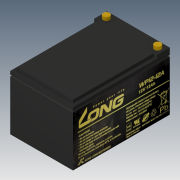
# Autodesk Inventor part: 800-10-ELECTRONICS-BATTERY-12V-12Ah
Saved by Autodesk Inventor 2018.2 (Build 222227000, 227)
## iProperties
Manager: feesmrt
Company: FRANC0R
Created: 2017-12-05
Part Number: 800-10-ELECTRONICS-BATTERY-12V-12Ah
Material: ABS-Kunststoff
Document SubType Name: Modeling
Designer: feesmrt
Density: 1.06 g/cm^3
Appearance: Glatt - schwarz
Project: Rescue Robot
Cost Center: -
Engineer: feesmrt
Authority: feesmrt
Description: Lead-Acid Battery WP12-12 12V 12Ah
Stock Number: 800-10-ELECTRONICS-BATTERY-12V-12Ah
Catalog Web Link: Reichelt
Vendor: https://www.reichelt.de/Blei-Vlies-Akkus-12V-Kung-Long/WP-12-12/3/index.html?ACTION=3&GROUPID=4232&ARTICLE=44421&START=0&OFFSET
Author: feesmrt
Subject: Rescue Robot
Title: Lead-Acid Battery WP12-12 12V 12Ah
Revision Number: 1
Autodesk Inventor part; units mm, degrees
ref_plane "YZ Plane" through (0, 0, 0) normal (1, 0, 0) x (0, 1, 0)
ref_plane "XZ Plane" through (0, 0, 0) normal (0, 1, 0) x (-1, 0, 0)
ref_plane "XY Plane" through (0, 0, 0) normal (0, 0, 1) x (1, 0, 0)
sketch "Skizze1" plane through (0, 0, 0) normal (0, 0, 1) x (1, 0, 0)
  line L0 (-49, -75.5) -> (49, -75.5)
  line L1 (49, -75.5) -> (49, 75.5)
  line L2 (49, 75.5) -> (-49, 75.5)
  line L3 (-49, 75.5) -> (-49, -75.5)
  line L4 (-49, -75.5) -> (49, 75.5) construction
  line L5 (49, -75.5) -> (-49, 75.5) construction
  point P0 (0, 0)
  dimension "d0" = 98
  dimension "d1" = 151
  constraints: 12 end point, 2 midpoint, 2 parallel, 1 horizontal, 1 perpendicular
  measures "d0" distance of L1.end L2.end
  measures "d1" distance of L0.end L1.end
extrude "Grundkörper" add sketch "Skizze1" along normal blind 83
chamfer "Fase" distance 2.5 angle 45 8 edges at (-49, 0, 83) (0, -75.5, 83) (49, 0, 83) (0, 75.5, 83) (0, -75.5, 0) (-49, 0, 0) (49, 0, 0) (0, 75.5, 0)
sketch "Skizze2" plane through (0, 0, 83) normal (0, 0, 1) x (1, 0, 0)
  line L0 (49, -75.5) -> (49, 75.5) projected
  line L1 (49, 75.5) -> (-49, 75.5) projected
  line L2 (-49, -75.5) -> (49, -75.5) projected
  line L3 (-49, 75.5) -> (-49, -75.5) projected
  point P0 (0, 0)
extrude "Cap" add sketch "Skizze2" along normal blind 10
sketch "Skizze3" plane through (0, 0, 93) normal (0, 0, 1) x (1, 0, 0)
  line L0 (44, 55.5) -> (-44, 55.5)
  line L1 (-44, 55.5) -> (-44, -70.5)
  line L2 (-44, -70.5) -> (44, -70.5)
  line L3 (44, -70.5) -> (44, 55.5)
  line L4 (0, 105.7) -> (0, -105.7) construction
  line L5 (49, -75.5) -> (49, 75.5) projected
  line L6 (-49, -75.5) -> (49, -75.5) projected
  line L7 (44, 55.5) -> (49, 55.5)
  line L8 (49, -75.5) -> (49, 75.5) projected
  line L9 (49, 55.5) -> (49, -75.5)
  line L10 (-49, 75.5) -> (-49, -75.5) projected
  line L11 (49, -75.5) -> (-49, -75.5)
  line L12 (-49, -75.5) -> (-49, 55.5)
  line L13 (-44, 55.5) -> (-49, 55.5)
  line L14 (-46.5, -73) -> (-46.5, 73) projected
  line L15 (49, 75.5) -> (-49, 75.5) projected
  point P0 (0, 0)
  dimension "d9" = 5
  dimension "d10" = 5
  dimension "d13" = 20
  constraints: 18 end point, 4 perpendicular, 2 parallel, 2 point on line, 1 collinear, 1 horizontal, 1 other
  measures "d9" distance between parallel lines of L5 L3
  measures "d10" distance between parallel lines of L6 L2
  measures "d13" distance between parallel lines of L15 L0
extrude "Absatz" cut sketch "Skizze3" against normal blind 5 contours L7 L5 L6 L10 L13 L1 L2 L3
sketch "Skizze4" plane through (0, 0, 93) normal (0, 0, 1) x (1, 0, 0)
  line L0 (44, 55.5) -> (49, 55.5) projected
  line L1 (49, 75.5) -> (-49, 75.5) projected
  line L2 (49, 55.5) -> (49, 75.5) projected
  line L3 (-49, 75.5) -> (-49, 55.5) projected
  line L4 (49, 55.5) -> (-49, 55.5)
  line L5 (-49, 75.5) -> (-49, -75.5) projected
  line L6 (-49, 65.5) -> (49, 65.5) construction
  line L7 (49, 75.5) -> (49, -75.5) projected
  line L8 (0, 105.7) -> (0, -105.7) construction
  circle A0 centre (40, 65.5) radius 5
  circle A1 centre (-40, 65.5) radius 5
  point P0 (0, 0)
  dimension "d14" = 10
  dimension "d15" = 80
  constraints: 4 end point, 4 point on line, 2 centre point, 1 equal radius, 1 horizontal, 1 symmetric about line
  measures "d14" diameter of A0
  measures "d15" distance of A1.centre A0.centre
extrude "Connectors" add sketch "Skizze4" along normal blind 5 contours A0 | A1
